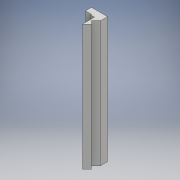
# Autodesk Inventor part: SlidingLock
Saved by Autodesk Inventor 2018 (Build 220112000, 112)
## iProperties
Created: 2019-10-04
Part Number: SlidingLock
Material: Generic
Document SubType Name: Modeling
Designer: Ivan
Density: 1 g/cm^3
Appearance: Default
Author: Ivan
Autodesk Inventor part; units mm, degrees
ref_plane "YZ Plane" through (0, 0, 0) normal (1, 0, 0) x (0, 1, 0)
ref_plane "XZ Plane" through (0, 0, 0) normal (0, 1, 0) x (-1, 0, 0)
ref_plane "XY Plane" through (0, 0, 0) normal (0, 0, 1) x (1, 0, 0)
sketch "Sketch1" plane through (0, 0, 0) normal (0, 0, 1) x (1, 0, 0)
  line L0 (0, -6) -> (0, -3) construction
  line L1 (2.25, -3.75) -> (0, -6) construction
  line L2 (2.25, -3.75) -> (0, -6)
  line L3 (0, -6) -> (0, -3)
  line L4 (0, -3) -> (0, 0)
  line L5 (0.75, -2.25) -> (3, 0) construction
  line L6 (2.25, -3.75) -> (0.75, -2.25)
  line L7 (3, 0) -> (0.75, -2.25)
  line L8 (0, 0) -> (3, 0)
  point P0 (0, -1.5)
  constraints: 18 end point, 2 collinear, 2 perpendicular, 2 vertical, 1 midpoint, 1 vertical alignment
extrude "Extrusion1" add sketch "Sketch1" along normal blind 63
sketch "Sketch2" plane through (0, 0, 0) normal (0, 1, 0) x (1, 0, 0)
  line L0 (0.75, -63) -> (3, -63) projected
  line L1 (3, -63) -> (-2, -63)
  line L2 (-2, -63) -> (-2, 0)
  line L3 (-2, 0) -> (3, 0)
  line L4 (3, 0) -> (3, -63)
  point P0 (0, 0)
  dimension "d2" = 5
  dimension "d3" = 63
  constraints: 8 end point, 2 parallel, 1 horizontal, 1 perpendicular
  measures "d2" distance between parallel lines of L2 L4
  measures "d3" distance between parallel lines of L3 L1
extrude "Extrusion2" add sketch "Sketch2" along normal blind 0.5
sketch "Sketch3" plane through (0, 0.5, 0) normal (0, 1, 0) x (1, 0, 0)
  line L0 (0.75, -63) -> (3, -63) projected
  line L1 (3, -63) -> (-5, -63)
  line L2 (-5, -63) -> (-5, 0)
  line L3 (-5, 0) -> (3, 0)
  line L4 (3, 0) -> (3, -63)
  point P0 (0, 0)
  dimension "d6" = 63
  dimension "d7" = 8
  constraints: 8 end point, 2 parallel, 1 horizontal, 1 perpendicular
  measures "d6" distance between parallel lines of L1 L3
  measures "d7" distance between parallel lines of L4 L2
extrude "Extrusion3" add sketch "Sketch3" along normal blind 3
body "Solid1"
